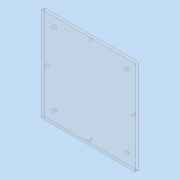
# Autodesk Inventor part: WaagePlexiOben2
Saved by Autodesk Inventor 2022 (Build 260153000, 153)
## iProperties
Created: 2021-12-03
Part Number: WaagePlexiOben2
Material: PET Plastic
Document SubType Name: Modeling
Designer: domin
Density: 1.541 g/cm^3
Appearance: Polycarbonate - Clear
Mass: 110.779 g
Surface Area: 366.745 cm^2
Volume: 71.8875 cm^3
Author: domin
Autodesk Inventor part; units mm, degrees
ref_plane "YZ Plane" through (0, 0, 0) normal (1, 0, 0) x (0, 1, 0)
ref_plane "XZ Plane" through (0, 0, 0) normal (0, 1, 0) x (-1, 0, 0)
ref_plane "XY Plane" through (0, 0, 0) normal (0, 0, 1) x (1, 0, 0)
sketch "Sketch1" plane through (0, 0, 0) normal (0, 0, 1) x (1, 0, 0)
  line L0 (-89, 89) -> (89, 89)
  line L1 (89, 89) -> (89, -89)
  line L2 (89, -89) -> (-89, -89)
  line L3 (-89, -89) -> (-89, 89)
  point P0 (0, 0)
  dimension "d33" = 178
  dimension "d34" = 89
  dimension "d35" = 89
  constraints: 8 end point, 2 parallel, 2 perpendicular, 1 horizontal
  measures "d33" distance between parallel lines of L1 L3
  measures "d34" distance from line of point (0, 0) L0
  measures "d35" distance from line of point (0, 0) L3
extrude "Extrusion1" add sketch "Sketch1" along normal blind 5
sketch "Sketch2" plane through (0, 0, 5) normal (0, 0, 1) x (1, 0, 0)
  circle A0 centre (-81.5, 0) radius 2
  circle A1 centre (81.5, 0) radius 2
  line L0 (-78.5, 36.125) -> (-78.5, 56.125) projected
  line L1 (78.5, 56.125) -> (78.5, 36.125) projected
  circle A2 centre (0, 81.5) radius 2
  circle A3 centre (0, -81.5) radius 2
  line L2 (36.125, 78.5) -> (56.125, 78.5) projected
  line L3 (56.125, -78.5) -> (36.125, -78.5) projected
  line L4 (-89, 89) -> (-89, -89) projected
  line L5 (89, 89) -> (-89, 89) projected
  line L6 (89, -89) -> (89, 89) projected
  line L7 (-89, -89) -> (89, -89) projected
  point P0 (0, 0)
  point P1 (-78.5, -56.125)
  point P2 (78.5, -56.125)
  point P3 (-56.125, 78.5)
  point P4 (-56.125, -78.5)
  dimension "d18" = 4
  dimension "d37" = 7.5
  dimension "d38" = 7.5
  dimension "d39" = 7.5
  dimension "d40" = 7.5
  constraints: 4 centre point, 3 equal radius, 2 horizontal alignment, 2 vertical alignment
  measures "d18" diameter of A0
  measures "d37" distance from line of A0.centre L4
  measures "d38" distance from line of L5 A2.centre
  measures "d39" distance from line of L6 A1.centre
  measures "d40" distance from line of L7 A3.centre
hole "Hole1" at (-81.5, 0, 5) at (0, 81.5, 5) at (81.5, 0, 5) at (0, -81.5, 5) direction (0, 0, -1) diameter 4 end through all
fillet "Fillet1" radius 2 4 edges at (-89, -89, 2.5) (-89, 89, 2.5) (89, -89, 2.5) (89, 89, 2.5)
sketch "Sketch3" plane through (0, 0, 5) normal (0, 0, 1) x (1, 0, 0)
  line L0 (68.475, -68.475) -> (-68.475, -68.475)
  line L1 (-68.475, -68.475) -> (-68.475, 68.475)
  line L2 (-68.475, 68.475) -> (68.475, 68.475)
  line L3 (68.475, 68.475) -> (68.475, -68.475)
  line L4 (68.475, -68.475) -> (-68.475, 68.475) construction
  line L5 (-68.475, -68.475) -> (68.475, 68.475) construction
  circle A0 centre (-68.475, 68.475) radius 4.875
  point P0 (0, 0)
  dimension "d31" = 136.95
  dimension "d32" = 9.75
  constraints: 12 end point, 2 midpoint, 2 parallel, 2 perpendicular, 1 centre point, 1 coincident, 1 horizontal
  measures "d31" distance of L1.end L2.end
  measures "d32" diameter of A0
hole "Hole2" at (-68.475, 68.475, 5) at (68.475, 68.475, 5) at (68.475, -68.475, 5) at (-68.475, -68.475, 5) direction (0, 0, -1) diameter 6 end through all
equation "\"d34\" = 0.5 * d33"
equation "\"d35\" = 0.5 * d33"
equation "\"d38\" = d37"
equation "\"d39\" = d37"
equation "\"d40\" = d37"
equation "\"d21\" = d18"
equation "\"d6\" = 0.5 * d3"
equation "\"d7\" = 0.5 * d2"
equation "\"d3\" = 157"
equation "\"d2\" = 157"
body "Solid1"
